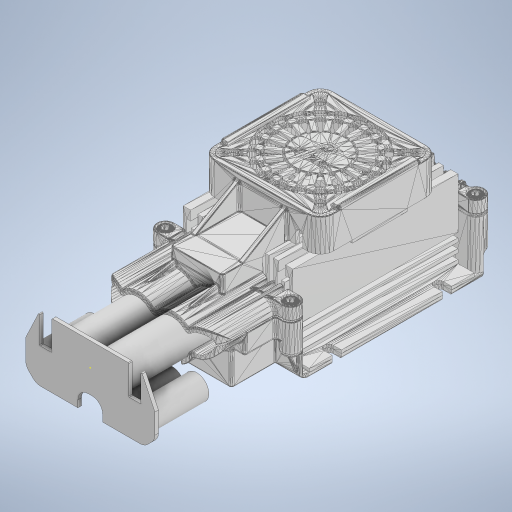
# Autodesk Inventor part: Mamba XLX ESC
Saved by Autodesk Inventor 2023 (Build 270158000, 158)
## iProperties
Created: 2022-07-14
Part Number: Mamba XLX ESC
Material: Generic
Document SubType Name: Modeling
Designer: justi
Density: 1 g/cm^3
Appearance: Default
Author: justi
Autodesk Inventor part; units mm, degrees
ref_plane "YZ Plane" through (0, 0, 0) normal (1, 0, 0) x (0, 1, 0)
ref_plane "XZ Plane" through (0, 0, 0) normal (0, 1, 0) x (-1, 0, 0)
ref_plane "XY Plane" through (0, 0, 0) normal (0, 0, 1) x (1, 0, 0)
sketch "Sketch1" plane through (-4.5, -9.15, 9.417) normal (0, -1, 0) x (1, 0, 0)
  point P0 (4.5, -9.417)
sketch "Sketch2" plane through (1.8079, 5.5858, 15) normal (0, 0, 1) x (1, 0, 0)
  line L0 (-1.8079, -5.5858) -> (-1.8079, -0.7733)
  circle A0 centre (-8.2214, -4.4747) radius 6.35
  circle A1 centre (4.6056, -4.4747) radius 6.35
  dimension "d0" = 12.7
  dimension "d1" = 6.4135
  dimension "d2" = 12.7
  dimension "d3" = 6.4135
  constraints: 2 centre point, 2 end point, 1 vertical
  measures "d0" diameter of A0
  measures "d1" distance from line of L0 A0.centre
  measures "d2" diameter of A1
  measures "d3" distance from line of L0 A1.centre
extrude "Extrusion1" add sketch "Sketch2" along normal mid plane 44.45
sketch "Sketch4" plane through (6.4135, 1.1111, 37.225) normal (0, 0, 1) x (1, 0, 0)
  circle A0 centre (3.175, -10.541) radius 4.445
  circle A1 centre (0, 0) radius 6.35 projected
  point P0 (-6.4135, -1.1111)
  dimension "d7" = 8.89
  dimension "d8" = 10.541
  dimension "d9" = 3.175
  constraints: 1 centre point
  measures "d7" diameter of A0
  measures "d8" vertical distance of A1.centre A0.centre
  measures "d9" horizontal distance of A1.centre A0.centre
sketch "Sketch5" plane through (-6.4135, 1.1111, 37.225) normal (0, 0, 1) x (1, 0, 0)
  circle A0 centre (-3.175, -10.541) radius 4.445
  circle A1 centre (0, 0) radius 6.35 projected
  point P0 (6.4135, -1.1111)
  dimension "d10" = 8.89
  dimension "d11" = 3.175
  dimension "d12" = 10.541
  constraints: 1 centre point
  measures "d10" diameter of A0
  measures "d11" horizontal distance of A1.centre A0.centre
  measures "d12" vertical distance of A1.centre A0.centre
extrude "Extrusion2" add sketch "Sketch4" against normal blind 19.05 contours A0
extrude "Extrusion3" add sketch "Sketch5" against normal blind 19.05 contours A0
sketch "Sketch6" plane through (-9.5885, -9.4299, 37.225) normal (0, 0, 1) x (1, 0, 0)
  circle A0 centre (-8.89, 2.54) radius 4.445
  circle A1 centre (0, 0) radius 4.445 projected
  line L0 (0, 0) -> (0, 2.54)
  point P0 (9.5885, 9.4299)
  dimension "d17" = 8.89
  dimension "d18" = 8.89
  dimension "d52" = 2.54
  dimension "d53" = 0
  constraints: 2 end point, 1 centre point, 1 vertical
  measures "d17" diameter of A0
  measures "d18" horizontal distance of L0.start A0.centre
  measures "d52" distance of L0.start L0.end
  measures "d53" vertical distance of A0.centre L0.end
extrude "Extrusion4" add sketch "Sketch6" against normal blind 19.05 contours A0
sketch "Sketch7" plane through (9.5885, -9.4299, 37.225) normal (0, 0, 1) x (1, 0, 0)
  circle A0 centre (8.89, 2.54) radius 4.445
  circle A1 centre (0, 0) radius 4.445 projected
  line L0 (0, 0) -> (0, 2.54)
  point P0 (-9.5885, 9.4299)
  dimension "d22" = 8.89
  dimension "d54" = 2.54
  dimension "d55" = 0
  constraints: 2 end point, 1 centre point, 1 vertical
  measures "d22" diameter of A0
  measures "d54" distance of L0.start L0.end
  measures "d55" vertical distance of A0.centre L0.end
extrude "Extrusion5" add sketch "Sketch7" against normal blind 19.05 contours A0
sketch "Sketch8" plane through (6.4135, 1.1111, 37.225) normal (0, 0, 1) x (1, 0, 0)
  line L0 (-7.62, -6.7786) -> (7.62, -6.7786)
  line L1 (7.62, -6.7786) -> (7.62, 7.1914)
  line L2 (7.62, 7.1914) -> (-7.62, 7.1914)
  line L3 (-7.62, 7.1914) -> (-7.62, -6.7786)
  line L4 (-7.62, -6.7786) -> (7.62, 7.1914) construction
  line L5 (7.62, -6.7786) -> (-7.62, 7.1914) construction
  point P0 (-6.4135, -1.1111)
  point P1 (0, 0.2064)
  dimension "d27" = 15.24
  dimension "d28" = 13.97
  constraints: 12 end point, 2 midpoint, 2 parallel, 1 horizontal, 1 perpendicular
  measures "d27" distance of L2.end L1.end
  measures "d28" distance of L0.end L1.end
sketch "Sketch9" plane through (-6.4135, 1.1111, 37.225) normal (0, 0, 1) x (1, 0, 0)
  line L0 (-7.62, -6.7768) -> (7.62, -6.7768)
  line L1 (7.62, -6.7768) -> (7.62, 7.1932)
  line L2 (7.62, 7.1932) -> (-7.62, 7.1932)
  line L3 (-7.62, 7.1932) -> (-7.62, -6.7768)
  line L4 (-7.62, -6.7768) -> (7.62, 7.1932) construction
  line L5 (7.62, -6.7768) -> (-7.62, 7.1932) construction
  point P0 (6.4135, -1.1111)
  point P1 (0, 0.2082)
  dimension "d29" = 15.24
  dimension "d30" = 13.97
  constraints: 12 end point, 2 midpoint, 2 parallel, 1 horizontal, 1 perpendicular
  measures "d29" distance of L2.end L1.end
  measures "d30" distance of L2.end L0.start
extrude "Extrusion6" add sketch "Sketch9" along normal blind 1.27
extrude "Extrusion7" add sketch "Sketch8" along normal blind 1.27
sketch "Sketch10" plane through (-6.4135, 1.1111, 38.495) normal (0, 0, 1) x (1, 0, 0)
  line L0 (-7.62, -9.6614) -> (20.447, -9.6614)
  line L1 (20.447, -9.6614) -> (20.447, 7.4393)
  line L2 (20.447, 7.4393) -> (-7.62, 7.4393)
  line L3 (-7.62, 7.4393) -> (-7.62, -9.6614)
  line L4 (-7.62, -9.6614) -> (20.447, 7.4393) construction
  line L5 (20.447, -9.6614) -> (-7.62, 7.4393) construction
  point P0 (6.4135, -1.1111)
  constraints: 12 end point, 2 midpoint, 2 parallel, 1 horizontal, 1 perpendicular
extrude "Extrusion8" add sketch "Sketch10" against normal blind 1.27
sketch "Sketch11" plane through (-6.4135, 1.1111, 38.495) normal (0, 0, 1) x (1, 0, 0)
  line L0 (-17.145, -16.0114) -> (1.905, -16.0114)
  line L1 (1.905, -16.0114) -> (1.905, -3.3114)
  line L2 (1.905, -3.3114) -> (-17.145, -3.3114)
  line L3 (-17.145, -3.3114) -> (-17.145, -16.0114)
  line L4 (-7.62, -9.6614) -> (-7.62, 7.4393) projected
  line L5 (-17.145, -16.0114) -> (1.905, -3.3114) construction
  line L6 (1.905, -16.0114) -> (-17.145, -3.3114) construction
  line L7 (10.922, -16.0114) -> (29.972, -16.0114)
  line L8 (29.972, -16.0114) -> (29.972, -3.3114)
  line L9 (29.972, -3.3114) -> (10.922, -3.3114)
  line L10 (10.922, -3.3114) -> (10.922, -16.0114)
  line L11 (20.447, -9.6614) -> (20.447, 7.4393) projected
  line L12 (10.922, -16.0114) -> (29.972, -3.3114) construction
  line L13 (29.972, -16.0114) -> (10.922, -3.3114) construction
  line L14 (-12.065, -3.3114) -> (-12.065, 7.4393)
  line L15 (24.892, -3.3114) -> (24.892, 7.4393)
  line L16 (24.892, 7.4393) -> (29.972, -3.3114)
  line L17 (-17.145, -3.3114) -> (-12.065, 7.4393)
  point P0 (6.4135, -1.1111)
  dimension "d37" = 19.05
  dimension "d38" = 12.7
  dimension "d39" = 19.05
  dimension "d40" = 12.7
  dimension "d41" = 5.08
  dimension "d42" = 5.08
  constraints: 32 end point, 4 midpoint, 4 parallel, 2 horizontal, 2 perpendicular, 2 point on line, 2 vertical
  measures "d37" distance of L2.end L1.end
  measures "d38" distance of L0.end L1.end
  measures "d39" distance of L9.end L8.end
  measures "d40" distance of L7.end L8.end
  measures "d41" distance from line of L2.end L14
  measures "d42" distance from line of L8.end L15
extrude "Extrusion9" add sketch "Sketch11" against normal blind 1.27
fillet "Fillet1" radius 0.254 2 edges at (-18.4785, 8.5503, 37.86) (18.4785, 8.5503, 37.86)
fillet "Fillet2" radius 0.254 6 edges at (-14.0335, 8.5503, 37.86) (-18.4785, -2.2003, 37.86) (-14.0335, -2.2003, 37.86) (14.0335, -2.2003, 37.86) (18.4785, -2.2003, 37.86) (14.0335, 8.5503, 37.86)
fillet "Fillet3" radius 3.81 4 edges at (-23.5585, -14.9003, 37.86) (23.5585, -14.9003, 37.86) (-4.5085, -8.5503, 37.86) (4.5085, -8.5503, 37.86)
sketch "Sketch13" plane through (-6.4135, 1.1111, 38.495) normal (0, 0, 1) x (1, 0, 0)
  point P0 (6.4135, -1.1111)
sketch "Sketch14" plane through (-6.4135, 1.1111, 38.495) normal (0, 0, 1) x (1, 0, 0)
  arc A0 (-17.145, -12.2014) -> (-13.335, -16.0114) centre (-13.335, -12.2014) ccw projected
  line L0 (-17.145, -12.2014) -> (-13.335, -16.0114)
  line L1 (-13.335, -16.0114) -> (-15.2586, -17.935)
  line L2 (-15.2586, -17.935) -> (-19.0686, -14.125)
  line L3 (-19.0686, -14.125) -> (-17.145, -12.2014)
  arc A1 (26.162, -16.0114) -> (29.972, -12.2014) centre (26.162, -12.2014) ccw projected
  line L4 (26.162, -16.0114) -> (29.972, -12.2014)
  line L5 (29.972, -12.2014) -> (31.5861, -13.8155)
  line L6 (31.5861, -13.8155) -> (27.7761, -17.6255)
  line L7 (27.7761, -17.6255) -> (26.162, -16.0114)
  point P0 (6.4135, -1.1111)
  constraints: 16 end point, 5 parallel, 2 perpendicular
extrude "Extrusion10" cut sketch "Sketch14" against normal blind 1.27 contours L0 A0 | L4 A1
fillet "Fillet4" radius 3.81 4 edges at (-23.5585, -11.0903, 37.86) (-19.7485, -14.9003, 37.86) (23.5585, -11.0903, 37.86) (19.7485, -14.9003, 37.86)
body "Solid1"
